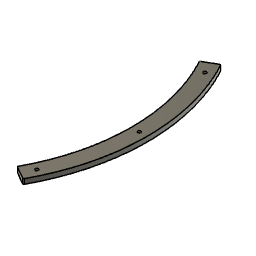
move_base_front_bumper_b (Autodesk Fusion 360 design; units mm, degrees)
Autodesk Fusion 360 part; units mm, degrees
note: some values were not read from the file. Set by a fixed rule: the direction of a hole.
sketch "スケッチ1" plane through (0, 0, 0) normal (0, 1, 0) x (1, 0, 0)
  arc A0 (181.8653, -105) -> (181.8653, 105) centre (0, 0) ccw
  line L0 (181.8653, 105) -> (0, 0)
  line L1 (0, 0) -> (181.8653, -105)
  line L2 (0, 0) -> (210, 0)
  arc A1 (168.0089, -97) -> (168.0089, 97) centre (0, 0) ccw
  line L3 (10, 0) -> (184.3138, 100.6401)
  line L4 (10, 0) -> (184.3138, -100.6401)
  arc A2 (183.0742, -85.3689) -> (183.0742, 85.3689) centre (0, 0) ccw
  line L5 (0, 0) -> (183.0742, 85.3689)
  line L6 (0, 0) -> (183.0742, -85.3689)
  point P0 (202, 0)
  dimension "d1" = 210
  dimension "d2" = 30
  dimension "d3" = 30
  dimension "d4" = 194
  dimension "d14" = 30
  dimension "d15" = 10
  dimension "d17" = 30
  dimension "d23" = 202
  dimension "d24" = 25
  dimension "d25" = 25
  constraint coincident A0.centre L0.end
  constraint coincident A0 L2.end
  constraint horizontal L2
  constraint coincident L0 A1.end
  constraint coincident L1 A1.start
  constraint coincident L2 L3.start
  constraint coincident A0 L3.end
  constraint coincident A0 L4.end
  constraint midpoint A2 P0
  measures "d1" radius of A0
  measures "d2" angle of L0 L2
  measures "d3" angle of L1 L2
  measures "d4" radius of A1
  measures "d14" angle of L2 L3
  measures "d15" distance of A0.centre L3.start
  measures "d17" angle of L2 L4
  measures "d23" radius of A2
  measures "d24" angle of L2 L5
  measures "d25" angle of L2 L6
extrude "押し出し1" add sketch "スケッチ1" along normal blind 5 contours A0 L2 A1 L4 A2 L6 | A0 L2 A1 L3 A2 L5 | L2 A1 A2 L6 | L2 A1 A2 L5
hole "穴1" at (183.0742, 0, 85.3689) at (202, 0, 0) at (183.0742, 0, -85.3689) direction (0, 1, 0) diameter 3.2 end through all
fillet "フィレット1" radius 1 4 edges at (184.3138, 2.5, 100.6401) (184.3138, 2.5, -100.6401) (170.4531, 2.5, 92.6377) (170.4531, 2.5, -92.6377)
